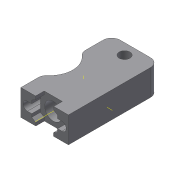
# Autodesk Inventor part: empty
Saved by Autodesk Inventor 2014 (Build 180170000, 170)
## iProperties
Created: 2015-04-13
Part Number: empty
Material: Generic
Document SubType Name: Modeling
Designer: Martin
Density: 1 g/cm^3
Appearance: Default
Mass: 0.578402 g
Surface Area: 7.54528 cm^2
Volume: 0.578402 cm^3
Author: Martin
Autodesk Inventor part; units mm, degrees
ref_plane "plane_support" through (-5.5, -8, -3) normal (0, -1, 0) x (1, 0, 0)
ref_plane "YZ Plane" through (0, 0, 0) normal (1, 0, 0) x (0, 1, 0)
ref_plane "XZ Plane" through (0, 0, 0) normal (0, 1, 0) x (-1, 0, 0)
sketch "Sketch14" plane through (0, 0, 0) normal (1, 0, 0) x (0, 1, 0)
  line L0 (-13.2, 0) -> (16.2, 0) projected
  line L1 (0, -4.2) -> (0, 4.2) projected
  line L2 (9, -3) -> (-9, -3)
  line L3 (-9, -3) -> (-9, 3)
  line L4 (-9, 3) -> (9, 3)
  line L5 (9, 3) -> (9, -3) construction
  line L6 (9, -3) -> (-9, 3) construction
  line L7 (-9, -3) -> (9, 3) construction
  line L8 (5.5, 3) -> (5.5, -3) construction
  line L9 (-6.5, 3) -> (-6.5, -3) construction
  arc A0 (9, -3) -> (9, 3) centre (9, 0) ccw
  circle A1 centre (9, 0) radius 1.25
  circle A2 centre (9, 0) radius 3 construction
  line L10 (6, 3) -> (6, -3) construction
  line L11 (12, -3) -> (9, -3)
  line L12 (9, -3) -> (9, 3)
  line L13 (9, 3) -> (12, 3)
  line L14 (12, 3) -> (12, -3)
  line L15 (12, -3) -> (9, 3) construction
  line L16 (9, -3) -> (12, 3) construction
  point P0 (0, 0)
  point P1 (0, 0)
  point P2 (10.5, 0)
  dimension "d72" = 6
  dimension "d73" = 12
  dimension "d74" = 2.5
  dimension "d75" = 2.5
  dimension "d76" = 0.5
  constraints: 30 end point, 7 point on line, 5 midpoint, 5 perpendicular, 4 parallel, 4 tangent, 3 centre point, 2 coincident, 2 horizontal, 2 point on circle, 1 concentric
  measures "d72" distance between parallel lines of L2 L4
  measures "d73" distance between parallel lines of L8 L9
  measures "d74" distance between parallel lines of L3 L9
  measures "d75" diameter of A1
  measures "d76" distance between parallel lines of L8 L10
extrude "ext_main" add sketch "Sketch14" along normal mid plane 11
sketch "sk_channel_nut" plane through (-5.5, -9, -3) normal (0, -1, 0) x (1, 0, 0)
  line L0 (-2.2, 3) -> (13.2, 3) projected
  line L1 (5.5, -1.8497) -> (5.5, 7.8497) projected
  circle A0 centre (5.5, 3) radius 2
  line L2 (5.5, 6.4641) -> (2.5, 4.7321)
  line L3 (2.5, 4.7321) -> (2.5, 1.2679)
  line L4 (2.5, 1.2679) -> (5.5, -0.4641)
  line L5 (5.5, -0.4641) -> (8.5, 1.2679)
  line L6 (8.5, 1.2679) -> (8.5, 4.7321)
  line L7 (8.5, 4.7321) -> (5.5, 6.4641)
  circle A1 centre (1.5, 3) radius 1
  circle A2 centre (9.5, 3) radius 1
  line L8 (1.5, 4) -> (2.5, 4)
  line L9 (1.5, 2) -> (2.5, 2)
  line L10 (9.5, 4) -> (8.5, 4)
  line L11 (9.5, 2) -> (8.5, 2)
  line L12 (11, 0) -> (0, 0) projected
  line L13 (11, 6) -> (0, 6) projected
  line L14 (0, 0) -> (0, 6) projected
  line L15 (3.4, 6) -> (3.4, 5.2517)
  line L16 (3.4456, 0.722) -> (3.4456, 0)
  line L17 (7.5544, 0.722) -> (7.5544, 0)
  line L18 (7.6, 6) -> (7.6, 5.2517)
  point P0 (5.5, 3)
  point P1 (2.5, 3)
  dimension "d85" = 4
  dimension "d86" = 120
  dimension "d87" = 6
  dimension "d88" = 2
  dimension "d95" = 4.2
  constraints: 28 end point, 17 point on line, 7 parallel, 5 equal length, 5 point on circle, 5 tangent, 3 centre point, 3 perpendicular, 1 coincident, 1 equal radius, 1 midpoint, 2 other
  measures "d85" diameter of A0
  measures "d86" angle of L7 L2
  measures "d87" distance between parallel lines of L3 L6
  measures "d88" diameter of A1
  measures "d95" distance between parallel lines of L18 L15
extrude "ext_cut_bottomscrews" cut sketch "sk_channel_nut" against normal blind 8 contours A2 L0 | A2 L11 L6 | L6 L10 A2 | L0 A2
extrude "ext_cut_bottom_nut" cut sketch "sk_channel_nut" against normal blind 2 contours L3 L2 L13 L1 A0 L0 | L0 A0 L1 L12 L4 L3 | L16 L4 L12 | L13 L2 L15 | A0 L1 L0 | L0 L1 A0 | L12 L1 L4 | L2 L1 L13 | L1 A0 L0 | L0 A0 L1 | L1 L13 L7 L6 L0 A0 | A0 L0 L6 L5 L12 L1 | L1 L12 L5 | L7 L13 L1 | L5 L17 L12 | L13 L18 L7
sketch "Sketch21" plane through (-5.5, 12, 3) normal (0, 0, 1) x (1, 0, 0)
  line L0 (11, 0) -> (11, -21) projected
  line L1 (0, 0) -> (11, 0) projected
  line L2 (0, -21) -> (0, 0) projected
  line L3 (3.4, -19) -> (7.6, -19) projected
  line L4 (5.5, 0) -> (5.5, -2.5815) construction
  arc A0 (2, 0) -> (0, -2) centre (2, -2) ccw
  arc A1 (11, -2) -> (9, 0) centre (9, -2) ccw
  circle A2 centre (5.5, -2.5) radius 1.25
  point P0 (5.5, -12)
  point P1 (5.5, -1.25)
  dimension "d106" = 2.5
  dimension "d105" = 2
  dimension "d107" = 1.25
  constraints: 6 point on line, 4 point on circle, 2 centre point, 2 end point, 2 symmetric about line, 2 tangent, 1 midpoint, 1 perpendicular, 1 vertical alignment, 3 other
  measures "d105" radius of A0
  measures "d107" distance from line of point (5.5, -1.25) L1
extrude "ext_cut_fronthole" cut sketch "Sketch21" against normal through all
extrude "ext_cut_channel" cut sketch "sk_channel_nut" against normal blind 16 contours A0 L1 L0 | L0 L1 A0 | L1 A0 L0 | L0 A0 L1
extrude "ext_cut_shortscrew" cut sketch "sk_channel_nut" against normal blind 4 contours A1 L0 | L0 A1 | A1 L8 L3 | L3 L9 A1
sketch "Sketch22" plane through (-2.1, -7, 3) normal (0, 0, 1) x (1, 0, 0)
  line L0 (-3.4, -2) -> (-3.4, 17) projected
  line L1 (0, -2) -> (-3.4, -2) projected
  line L2 (-3.4, 12) -> (-3.4, 3)
  arc A0 (-3.4, 3) -> (-3.4, 12) centre (-6.2, 7.5) ccw
  line L3 (-3.4, 7.5) -> (-0.9, 7.5) construction
  point P0 (2.1, 7)
  dimension "d112" = 5
  dimension "d113" = 9
  dimension "d119" = 2.5
  constraints: 4 end point, 3 point on circle, 2 point on line, 1 centre point, 1 collinear, 1 midpoint
  measures "d112" distance from line of L1 L2.end
  measures "d113" distance of L2.end L2.start
  measures "d119" distance of L3.start L3.end
extrude "ext_cut_cutway" cut sketch "Sketch22" against normal through all
fillet "Fillet1" radius 2 2 edges at (-5.5, 5, 0) (-5.5, -4, 0)
sketch "Sketch19" plane through (-5.5, -8, -3) normal (0, -1, 0) x (1, 0, 0)
  line L0 (3.4, 6) -> (7.6, 6) projected
  line L1 (3.4, 5.2517) -> (3.4, 6) projected
  line L2 (2.5, 4.7321) -> (3.4, 5.2517) projected
  line L3 (2.5, 1.2679) -> (2.5, 2) projected
  line L4 (3.4456, 0.722) -> (2.5, 1.2679) projected
  line L5 (3.4456, 0) -> (3.4456, 0.722) projected
  line L6 (7.5544, 0) -> (3.4456, 0) projected
  line L7 (7.5544, 0.722) -> (7.5544, 0) projected
  line L8 (8.5, 1.2679) -> (7.5544, 0.722) projected
  line L9 (8.5, 2) -> (8.5, 1.2679) projected
  line L10 (8.5, 4) -> (8.5, 2) projected
  line L11 (8.5, 4.7321) -> (8.5, 4) projected
  line L12 (7.6, 5.2517) -> (8.5, 4.7321) projected
  line L13 (7.6, 6) -> (7.6, 5.2517) projected
  circle A0 centre (5.5, 3) radius 2 projected
  line L14 (3.8, 5.675) -> (7.275, 5.675) construction
  line L15 (7.275, 5.675) -> (7.275, 5.064)
  line L16 (7.275, 5.064) -> (8.175, 4.5444)
  line L17 (8.175, 4.5444) -> (8.175, 4)
  line L18 (8.175, 4) -> (8.175, 2)
  line L19 (8.175, 2) -> (8.175, 1.4556)
  line L20 (8.175, 1.4556) -> (7.2294, 0.9097)
  line L21 (7.2294, 0.9097) -> (7.2294, 0.325)
  line L22 (7.2294, 0.325) -> (3.7706, 0.325) construction
  line L23 (3.7706, 0.325) -> (3.7706, 0.9097)
  line L24 (3.7706, 0.9097) -> (2.9, 1.4123)
  line L25 (2.9, 1.4123) -> (2.9, 2)
  line L26 (2.9, 2) -> (2.9, 4)
  line L27 (2.9, 4) -> (2.9, 4.5011)
  line L28 (2.9, 4.5011) -> (3.8, 5.0207)
  line L29 (3.8, 5.0207) -> (3.8, 5.675)
  line L30 (3.8, 5.675) -> (7.275, 5.675)
  line L31 (7.275, 5.675) -> (7.275, 6)
  line L32 (7.275, 6) -> (3.8, 6)
  line L33 (3.8, 6) -> (3.8, 5.675)
  line L34 (3.7706, 0.325) -> (7.2294, 0.325)
  line L35 (7.2294, 0.325) -> (7.2294, 0)
  line L36 (7.2294, 0) -> (3.7706, 0)
  line L37 (3.7706, 0) -> (3.7706, 0.325)
  line L38 (2.5, 2) -> (2.5, 4) projected
  line L39 (2.5, 4) -> (2.5, 4.7321) projected
  point P0 (5.5, 3)
  dimension "d97" = 0.4
  constraints: 48 end point, 6 equal length, 2 collinear, 2 perpendicular, 12 other
  measures "d97" horizontal distance of L14.start L0.start
equation "\"d73\" = linact_rod_effective_length"
equation "\"d74\" = nut_m3_thickness_max"
equation "\"d75\" = screw_m2_bore_loose"
equation "\"d87\" = nut_m3_width_acrossflats"
equation "\"d88\" = screw_m2_bore_selfthreading"
equation "\"d95\" = 0.7 * nut_m3_width_acrossflats"
equation "\"d93\" = 0.8 * nut_m3_thickness_max"
equation "\"d106\" = screw_m2_bore_loose"
equation "\"d107\" = 0.5 * screw_m2_bore_loose"
equation "\"d97\" = print_support_z_clearance"
equation "\"d96\" = print_support_xy_clearance"
equation "\"linact_rod_effective_length\" = 12"
equation "\"nut_m3_thickness_max\" = 2.5"
equation "\"screw_m2_bore_loose\" = 2.5"
equation "\"nut_m3_width_acrossflats\" = 6"
equation "\"screw_m2_bore_selfthreading\" = 2"
equation "\"print_support_z_clearance\" = 0.4"
equation "\"print_support_xy_clearance\" = 1"
body "Solid3"
